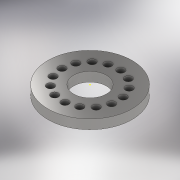
# Autodesk Inventor part: Orifice Plate
Saved by Autodesk Inventor 2021 (Build 250183000, 183)
## iProperties
Created: 2022-07-06
Part Number: Orifice Plate
Material: Stainless Steel
Document SubType Name: Modeling
Designer: pc
Density: 8 g/cm^3
Appearance: Semi-Polished
Mass: 491.031 g
Surface Area: 202.868 cm^2
Volume: 61.3789 cm^3
Author: pc
Autodesk Inventor part; units mm, degrees
ref_plane "YZ Plane" through (0, 0, 0) normal (1, 0, 0) x (0, 1, 0)
ref_plane "XZ Plane" through (0, 0, 0) normal (0, 1, 0) x (-1, 0, 0)
ref_plane "XY Plane" through (0, 0, 0) normal (0, 0, 1) x (1, 0, 0)
sketch "Sketch1" plane through (0, 0, 0) normal (0, 1, 0) x (-1, 0, 0)
  circle A0 centre (0, 0) radius 45
  dimension "d1" = 90
  constraints: 1 centre point, 1 coincident
  measures "d1" diameter of A0
extrude "Extrusion1" add sketch "Sketch1" along normal blind 10
sketch "Sketch2" plane through (0, 10, 0) normal (0, 1, 0) x (1, 0, 0)
  circle A0 centre (0, 0) radius 16
  dimension "d4" = 32
  constraints: 1 centre point, 1 coincident
  measures "d4" diameter of A0
hole "Hole1" at (0, 10, 0) direction (0, -1, 0) diameter 35 end through all
sketch "Sketch4" plane through (0, 10, 0) normal (0, 1, 0) x (1, 0, 0)
  point P0 (0, 0)
sketch "Sketch5" plane through (0, 10, 0) normal (0, 1, 0) x (1, 0, 0)
  circle A0 centre (-30, 0) radius 4
  circle A1 centre (-27.4064, -12.2021) radius 4
  circle A2 centre (-20.0739, -22.2943) radius 4
  circle A3 centre (-9.2705, -28.5317) radius 4
  circle A4 centre (3.1359, -29.8357) radius 4
  circle A5 centre (15, -25.9808) radius 4
  circle A6 centre (24.2705, -17.6336) radius 4
  circle A7 centre (29.3444, -6.2374) radius 4
  circle A8 centre (29.3444, 6.2374) radius 4
  circle A9 centre (24.2705, 17.6336) radius 4
  circle A10 centre (15, 25.9808) radius 4
  circle A11 centre (3.1359, 29.8357) radius 4
  circle A12 centre (-9.2705, 28.5317) radius 4
  circle A13 centre (-20.0739, 22.2943) radius 4
  circle A14 centre (-27.4064, 12.2021) radius 4
  point P0 (0, 0)
  dimension "d29" = 8
  dimension "d30" = 30
  dimension "d33" = 360
  constraints: 15 centre point, 31 other
  measures "d29" diameter of A0
  measures "d30" distance of A0.centre point (0, 0)
hole "Hole3" at (-27.4064, 10, 12.2021) at (-30, 10, 0) at (-27.4064, 10, -12.2021) at (-20.0739, 10, -22.2943) at (-9.2705, 10, -28.5317) at (3.1359, 10, -29.8357) at (15, 10, -25.9808) at (24.2705, 10, -17.6336) at (29.3444, 10, -6.2374) at (29.3444, 10, 6.2374) at (24.2705, 10, 17.6336) at (15, 10, 25.9808) at (3.1359, 10, 29.8357) at (-9.2705, 10, 28.5317) at (-20.0739, 10, 22.2943) direction (0, -1, 0) diameter 8 end through all
sketch "Sketch7" plane through (0, 10, 0) normal (0, 1, 0) x (1, 0, 0)
  point P0 (0, 0)
body "Solid1"
